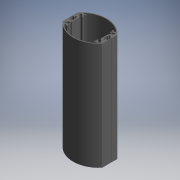
# Autodesk Inventor part: Funktionsprofil_LZ80
Saved by Autodesk Inventor 2017.3 (Build 213256000, 256)
## iProperties
Part Number: Funktionsprofil_LZ80
Material: Generic
Catalog Web Link: www.cadenas.de
Description: LZ80 Funktionsprofil-Bauteil LZ80
Vendor: ROSEKRIEGER
Document SubType Name: Modeling
Designer: partserver
Manufacturer: ROSEKRIEGER
Mass: 502.923 g
Surface Area: 2815.19 cm^2
Volume: 502.923 cm^3
Density: 1 g/cm^3
Appearance: PSOLRGB-128-128-128
Category: PARTsolutions
Company: ROSEKRIEGER
Title: Funktionsprofil_LZ80
Author: Cadenas PARTsolutions
Comments: Bauteil LZ80
PSOL_IDENT_0: {$CADENAS_DATA\23d-libs\rose_krieger\linearkomponenten\pool_lineartechnik\_hubsaeule_zyliinder\elekt
PSOL_IDENT_1: rozylinder\elekzyl_lz80\lz80_funktionsprofil.prj},194 {VTYP=3D},{NB=Funktionsprofil_LZ80},{LINA=Funk
PSOL_IDENT_2: tionsprofil_LZ80},{NN=LZ80 Funktionsprofil},{DATE=02.12.2020 11:16:39},{GEOMDATE=12.12.2006 09:47:00
PSOL_IDENT_3: },{VERSION=},{LINEID=10},{WBVAR=},{WBNUMERIC=}  {NB=Funktionsprofil_LZ80},{LINA=Funktionsprofil_LZ80
PSOL_IDENT_4: },{KT=DUMMY},{IDNR=},{ARTIKEL=Funktionsprofil_LZ80},{LAENGE=305.000}
NB: Funktionsprofil_LZ80
NN: LZ80 Funktionsprofil
NT: Bauteil LZ80
NBSYN: $ARTIKEL.
LINA: Funktionsprofil_LZ80
CATALOG: RK Rose+Krieger
ARTIKEL: Funktionsprofil_LZ80
LAENGE: 305
SUPPLIER: ROSEKRIEGER
ARTICLENO: Funktionsprofil_LZ80
BOMINFO: Funktionsprofil_LZ80
CREATOR: CADENAS GmbH
Autodesk Inventor part; units mm, degrees
ref_plane "YZ Plane" through (0, 0, 0) normal (1, 0, 0) x (0, 1, 0)
ref_plane "XZ Plane" through (0, 0, 0) normal (0, 1, 0) x (-1, 0, 0)
ref_plane "XY Plane" through (0, 0, 0) normal (0, 0, 1) x (1, 0, 0)
sketch "Skizze_1" plane through (0, 0, 0) normal (0, 0, 1) x (1, 0, 0)
  arc A0 (-56, 6.3) -> (-55.7, 6) centre (-55.7, 6.3) ccw
  line L0 (-55.7, 6) -> (-55.7, -6)
  arc A1 (-55.7, -6) -> (-56, -6.3) centre (-55.7, -6.3) ccw
  line L1 (-56, -6.3) -> (-56, -21.4274)
  arc A2 (-56, -21.4274) -> (-55.9534, -21.5558) centre (-55.8, -21.4274) ccw
  arc A3 (-55.9534, -21.5558) -> (55.9534, -21.5558) centre (0, 25.2452) ccw
  arc A4 (55.9534, -21.5558) -> (56, -21.4274) centre (55.8, -21.4274) ccw
  line L2 (56, -21.4274) -> (56, -6.3)
  arc A5 (56, -6.3) -> (55.7, -6) centre (55.7, -6.3) ccw
  line L3 (55.7, -6) -> (55.7, 6)
  arc A6 (55.7, 6) -> (56, 6.3) centre (55.7, 6.3) ccw
  line L4 (56, 6.3) -> (56, 21.4274)
  arc A7 (56, 21.4274) -> (55.9534, 21.5558) centre (55.8, 21.4274) ccw
  arc A8 (55.9534, 21.5558) -> (-55.9534, 21.5558) centre (0, -25.2452) ccw
  arc A9 (-55.9534, 21.5558) -> (-56, 21.4274) centre (-55.8, 21.4274) ccw
  line L5 (-56, 21.4274) -> (-56, 6.3)
  line L6 (43.5, 4.3) -> (43.5, -4.3)
  arc A10 (43.5, -4.3) -> (43.7, -4.5) centre (43.7, -4.3) ccw
  line L7 (43.7, -4.5) -> (45.3, -4.5)
  arc A11 (45.5, -4.7) -> (45.3, -4.5) centre (45.3, -4.7) ccw
  line L8 (45.5, -4.7) -> (45.5, -8.55)
  arc A12 (45.5, -8.55) -> (45.7, -8.75) centre (45.7, -8.55) ccw
  line L9 (45.7, -8.75) -> (49.8, -8.75)
  arc A13 (49.8, -8.75) -> (50, -8.55) centre (49.8, -8.55) ccw
  line L10 (50, -8.55) -> (50, -5.3)
  arc A14 (50.2, -5.1) -> (50, -5.3) centre (50.2, -5.3) ccw
  line L11 (50.2, -5.1) -> (54.3, -5.1)
  line L12 (54.3, -5.1) -> (54.3, 5.1)
  line L13 (54.3, 5.1) -> (50.2, 5.1)
  arc A15 (50, 5.3) -> (50.2, 5.1) centre (50.2, 5.3) ccw
  line L14 (50, 5.3) -> (50, 8.55)
  arc A16 (50, 8.55) -> (49.8, 8.75) centre (49.8, 8.55) ccw
  line L15 (49.8, 8.75) -> (45.7, 8.75)
  arc A17 (45.7, 8.75) -> (45.5, 8.55) centre (45.7, 8.55) ccw
  line L16 (45.5, 8.55) -> (45.5, 4.7)
  arc A18 (45.3, 4.5) -> (45.5, 4.7) centre (45.3, 4.7) ccw
  line L17 (45.3, 4.5) -> (43.7, 4.5)
  arc A19 (43.7, 4.5) -> (43.5, 4.3) centre (43.7, 4.3) ccw
  arc A20 (-49.7006, -19.3988) -> (-49.8855, -21.512) centre (-48.7365, -20.5478) ccw
  line L18 (-49.8855, -21.512) -> (-49.307, -22.2014)
  arc A21 (-49.307, -22.2014) -> (-47.1938, -22.3863) centre (-48.1579, -21.2373) ccw
  line L19 (-47.1938, -22.3863) -> (-46.2621, -21.6046)
  arc A22 (-46.0758, -21.5663) -> (-46.2621, -21.6046) centre (-46.1335, -21.7578) ccw
  arc A23 (-46.0758, -21.5663) -> (-41.2808, -17.7918) centre (-45, -18) ccw
  arc A24 (-40.8684, -17.2715) -> (-41.2808, -17.7918) centre (-40.7816, -17.7639) ccw
  line L20 (-40.8684, -17.2715) -> (-39.4487, -17.0211)
  arc A25 (-38.275, -18.007) -> (-39.4487, -17.0211) centre (-39.275, -18.006) ccw
  arc A26 (-39.5342, -21.918) -> (-38.275, -18.007) centre (-45, -18) ccw
  arc A27 (-39.5342, -21.918) -> (-39.2504, -23.9646) centre (-38.3151, -22.7919) ccw
  arc A28 (-39.2504, -23.9646) -> (-37.7262, -25.1426) centre (0, 25.2452) ccw
  arc A29 (-39.5242, -27.5441) -> (-37.7262, -25.1426) centre (-38.6252, -26.3434) ccw
  arc A30 (-41.823, -25.7421) -> (-39.5242, -27.5441) centre (0, 25.2452) ccw
  arc A31 (-41.823, -25.7421) -> (-44.677, -29.2213) centre (-43.25, -27.4817) ccw
  arc A32 (-44.677, -29.2213) -> (44.677, -29.2213) centre (0, 25.2452) ccw
  arc A33 (44.677, -29.2213) -> (41.823, -25.7421) centre (43.25, -27.4817) ccw
  arc A34 (39.5242, -27.5441) -> (41.823, -25.7421) centre (0, 25.2452) ccw
  arc A35 (37.7262, -25.1426) -> (39.5242, -27.5441) centre (38.6252, -26.3434) ccw
  arc A36 (37.7262, -25.1426) -> (39.2504, -23.9646) centre (0, 25.2452) ccw
  arc A37 (39.2504, -23.9646) -> (39.5342, -21.918) centre (38.3151, -22.7919) ccw
  arc A38 (38.275, -18.007) -> (39.5342, -21.918) centre (45, -18) ccw
  arc A39 (39.4487, -17.0211) -> (38.275, -18.007) centre (39.275, -18.006) ccw
  line L21 (39.4487, -17.0211) -> (40.8684, -17.2715)
  arc A40 (41.2808, -17.7918) -> (40.8684, -17.2715) centre (40.7816, -17.7639) ccw
  arc A41 (41.2808, -17.7918) -> (46.0758, -21.5663) centre (45, -18) ccw
  arc A42 (46.2621, -21.6046) -> (46.0758, -21.5663) centre (46.1335, -21.7578) ccw
  line L22 (46.2621, -21.6046) -> (47.1938, -22.3863)
  arc A43 (47.1938, -22.3863) -> (49.307, -22.2014) centre (48.1579, -21.2373) ccw
  line L23 (49.307, -22.2014) -> (49.8855, -21.512)
  arc A44 (49.8855, -21.512) -> (49.7006, -19.3988) centre (48.7365, -20.5478) ccw
  line L24 (49.7006, -19.3988) -> (48.7689, -18.617)
  arc A45 (48.6989, -18.4401) -> (48.7689, -18.617) centre (48.8975, -18.4638) ccw
  arc A46 (48.6989, -18.4401) -> (43.942, -14.4284) centre (45, -18) ccw
  arc A47 (43.3, -13.949) -> (43.942, -14.4284) centre (43.8, -13.949) ccw
  line L25 (43.3, -13.949) -> (43.3, -11.75)
  arc A48 (43.3, -11.75) -> (42.8, -11.25) centre (42.8, -11.75) ccw
  line L26 (42.8, -11.25) -> (42.5, -11.25)
  arc A49 (41, -9.75) -> (42.5, -11.25) centre (42.5, -9.75) ccw
  line L27 (41, -9.75) -> (41, 9.75)
  arc A50 (42.5, 11.25) -> (41, 9.75) centre (42.5, 9.75) ccw
  line L28 (42.5, 11.25) -> (42.8, 11.25)
  arc A51 (42.8, 11.25) -> (43.3, 11.75) centre (42.8, 11.75) ccw
  line L29 (43.3, 11.75) -> (43.3, 13.949)
  arc A52 (43.942, 14.4284) -> (43.3, 13.949) centre (43.8, 13.949) ccw
  arc A53 (43.942, 14.4284) -> (48.6989, 18.4401) centre (45, 18) ccw
  arc A54 (48.7689, 18.617) -> (48.6989, 18.4401) centre (48.8975, 18.4638) ccw
  line L30 (48.7689, 18.617) -> (49.7006, 19.3988)
  arc A55 (49.7006, 19.3988) -> (49.8855, 21.512) centre (48.7365, 20.5478) ccw
  line L31 (49.8855, 21.512) -> (49.307, 22.2014)
  arc A56 (49.307, 22.2014) -> (47.1938, 22.3863) centre (48.1579, 21.2373) ccw
  line L32 (47.1938, 22.3863) -> (46.2621, 21.6046)
  arc A57 (46.0758, 21.5663) -> (46.2621, 21.6046) centre (46.1335, 21.7578) ccw
  arc A58 (46.0758, 21.5663) -> (41.2808, 17.7918) centre (45, 18) ccw
  arc A59 (40.8684, 17.2715) -> (41.2808, 17.7918) centre (40.7816, 17.7639) ccw
  line L33 (40.8684, 17.2715) -> (39.4487, 17.0211)
  arc A60 (38.275, 18.007) -> (39.4487, 17.0211) centre (39.275, 18.006) ccw
  arc A61 (39.5342, 21.918) -> (38.275, 18.007) centre (45, 18) ccw
  arc A62 (39.5342, 21.918) -> (39.2504, 23.9646) centre (38.3151, 22.7919) ccw
  arc A63 (39.2504, 23.9646) -> (37.7262, 25.1426) centre (0, -25.2452) ccw
  arc A64 (39.5242, 27.5441) -> (37.7262, 25.1426) centre (38.6252, 26.3434) ccw
  arc A65 (41.823, 25.7421) -> (39.5242, 27.5441) centre (0, -25.2452) ccw
  arc A66 (41.823, 25.7421) -> (44.677, 29.2213) centre (43.25, 27.4817) ccw
  arc A67 (44.677, 29.2213) -> (0, 45.2008) centre (0, -25.2452) ccw
  arc A68 (0, 45.2008) -> (-44.677, 29.2213) centre (0, -25.2452) ccw
  arc A69 (-44.677, 29.2213) -> (-41.823, 25.7421) centre (-43.25, 27.4817) ccw
  arc A70 (-39.5242, 27.5441) -> (-41.823, 25.7421) centre (0, -25.2452) ccw
  arc A71 (-37.7261, 25.1426) -> (-39.5242, 27.5441) centre (-38.6252, 26.3434) ccw
  arc A72 (-37.7261, 25.1426) -> (-39.2504, 23.9646) centre (0, -25.2452) ccw
  arc A73 (-39.2504, 23.9646) -> (-39.5342, 21.918) centre (-38.3151, 22.7919) ccw
  arc A74 (-38.275, 18.007) -> (-39.5342, 21.918) centre (-45, 18) ccw
  arc A75 (-39.4487, 17.0211) -> (-38.275, 18.007) centre (-39.275, 18.006) ccw
  line L34 (-39.4487, 17.0211) -> (-40.8684, 17.2715)
  arc A76 (-41.2808, 17.7918) -> (-40.8684, 17.2715) centre (-40.7816, 17.7639) ccw
  arc A77 (-41.2808, 17.7918) -> (-46.0758, 21.5663) centre (-45, 18) ccw
  arc A78 (-46.2621, 21.6046) -> (-46.0758, 21.5663) centre (-46.1335, 21.7578) ccw
  line L35 (-46.2621, 21.6046) -> (-47.1938, 22.3863)
  arc A79 (-47.1938, 22.3863) -> (-49.307, 22.2014) centre (-48.1579, 21.2373) ccw
  line L36 (-49.307, 22.2014) -> (-49.8855, 21.512)
  arc A80 (-49.8855, 21.512) -> (-49.7006, 19.3988) centre (-48.7365, 20.5478) ccw
  line L37 (-49.7006, 19.3988) -> (-48.7689, 18.617)
  arc A81 (-48.6989, 18.4401) -> (-48.7689, 18.617) centre (-48.8975, 18.4638) ccw
  arc A82 (-48.6989, 18.4401) -> (-43.942, 14.4284) centre (-45, 18) ccw
  arc A83 (-43.3, 13.949) -> (-43.942, 14.4284) centre (-43.8, 13.949) ccw
  line L38 (-43.3, 13.949) -> (-43.3, 11.75)
  arc A84 (-43.3, 11.75) -> (-42.8, 11.25) centre (-42.8, 11.75) ccw
  line L39 (-42.8, 11.25) -> (-42.5, 11.25)
  arc A85 (-41, 9.75) -> (-42.5, 11.25) centre (-42.5, 9.75) ccw
  line L40 (-41, 9.75) -> (-41, -9.75)
  arc A86 (-42.5, -11.25) -> (-41, -9.75) centre (-42.5, -9.75) ccw
  line L41 (-42.5, -11.25) -> (-42.8, -11.25)
  arc A87 (-42.8, -11.25) -> (-43.3, -11.75) centre (-42.8, -11.75) ccw
  line L42 (-43.3, -11.75) -> (-43.3, -13.949)
  arc A88 (-43.942, -14.4284) -> (-43.3, -13.949) centre (-43.8, -13.949) ccw
  arc A89 (-43.942, -14.4284) -> (-48.6989, -18.4401) centre (-45, -18) ccw
  arc A90 (-48.7689, -18.617) -> (-48.6989, -18.4401) centre (-48.8975, -18.4638) ccw
  line L43 (-48.7689, -18.617) -> (-49.7006, -19.3988)
  line L44 (-54.3, 5.1) -> (-54.3, -5.1)
  line L45 (-54.3, -5.1) -> (-50.2, -5.1)
  arc A91 (-50, -5.3) -> (-50.2, -5.1) centre (-50.2, -5.3) ccw
  line L46 (-50, -5.3) -> (-50, -8.55)
  arc A92 (-50, -8.55) -> (-49.8, -8.75) centre (-49.8, -8.55) ccw
  line L47 (-49.8, -8.75) -> (-45.7, -8.75)
  arc A93 (-45.7, -8.75) -> (-45.5, -8.55) centre (-45.7, -8.55) ccw
  line L48 (-45.5, -8.55) -> (-45.5, -4.7)
  arc A94 (-45.3, -4.5) -> (-45.5, -4.7) centre (-45.3, -4.7) ccw
  line L49 (-45.3, -4.5) -> (-43.7, -4.5)
  arc A95 (-43.7, -4.5) -> (-43.5, -4.3) centre (-43.7, -4.3) ccw
  line L50 (-43.5, -4.3) -> (-43.5, 4.3)
  arc A96 (-43.5, 4.3) -> (-43.7, 4.5) centre (-43.7, 4.3) ccw
  line L51 (-43.7, 4.5) -> (-45.3, 4.5)
  arc A97 (-45.5, 4.7) -> (-45.3, 4.5) centre (-45.3, 4.7) ccw
  line L52 (-45.5, 4.7) -> (-45.5, 8.55)
  arc A98 (-45.5, 8.55) -> (-45.7, 8.75) centre (-45.7, 8.55) ccw
  line L53 (-45.7, 8.75) -> (-49.8, 8.75)
  arc A99 (-49.8, 8.75) -> (-50, 8.55) centre (-49.8, 8.55) ccw
  line L54 (-50, 8.55) -> (-50, 5.3)
  arc A100 (-50.2, 5.1) -> (-50, 5.3) centre (-50.2, 5.3) ccw
  line L55 (-50.2, 5.1) -> (-54.3, 5.1)
  constraints: 202 point on circle, 112 end point, 101 centre point
extrude "Extrusion1" add sketch "Skizze_1" along normal blind 305
ref_plane "EPDECKEL_XY" through (0, 0, 305) normal (0, 0, 1) x (1, 0, 0)
ref_plane "EPDECKEL_YZ" through (0, 0, 305) normal (1, 0, 0) x (0, 1, 0)
ref_plane "EPDECKEL_ZX" through (0, 0, 305) normal (0, 1, 0) x (0, 0, 1)
ref_plane "EPGEHAEUSE_XY" through (0, 0, 0) normal (0, 0, 1) x (1, 0, 0)
ref_plane "EPGEHAEUSE_YZ" through (0, 0, 0) normal (1, 0, 0) x (0, 1, 0)
ref_plane "EPGEHAEUSE_ZX" through (0, 0, 0) normal (0, 1, 0) x (0, 0, 1)
body "Solid1"
